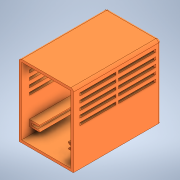
# Autodesk Inventor part: Back
Saved by Autodesk Inventor 2022 (Build 260153000, 153)
## iProperties
Created: 2022-01-12
Part Number: Back
Material: PLA Plastic
Document SubType Name: Modeling
Designer: chad
Density: 0.25 g/cm^3
Appearance: Generic(1)
Author: chad
Autodesk Inventor part; units mm, degrees
ref_plane "YZ Plane" through (0, 0, 0) normal (1, 0, 0) x (0, 1, 0)
ref_plane "XZ Plane" through (0, 0, 0) normal (0, 1, 0) x (-1, 0, 0)
ref_plane "XY Plane" through (0, 0, 0) normal (0, 0, 1) x (1, 0, 0)
sketch "Sketch1" plane through (0, 0, 0) normal (0, 0, 1) x (1, 0, 0)
  line L0 (0, 0) -> (42.2, 0)
  line L1 (42.2, 0) -> (42.2, 56.2)
  line L2 (42.2, 56.2) -> (0, 56.2)
  line L3 (0, 56.2) -> (0, 0)
  line L4 (17.1, 5) -> (25.1, 5) construction
  line L5 (17.1, 2.75) -> (25.1, 2.75)
  line L6 (25.1, 7.25) -> (17.1, 7.25)
  arc A0 (17.1, 7.25) -> (17.1, 2.75) centre (17.1, 5) ccw
  arc A1 (25.1, 2.75) -> (25.1, 7.25) centre (25.1, 5) ccw
  line L7 (21.1, 5) -> (29.1, 5) construction
  dimension "d0" = 42.2
  dimension "d1" = 56.2
  dimension "d2" = 4
  dimension "d3" = 0
  dimension "d4" = 4.5
  dimension "d91" = 21.1
  dimension "d92" = 5
  constraints: 18 end point, 4 point on circle, 4 tangent, 3 horizontal, 3 parallel, 2 centre point, 1 collinear, 1 midpoint, 1 perpendicular
  measures "d0" distance of L2.end L1.end
  measures "d1" distance of L1.end L0.end
  measures "d2" distance of L7.start L4.end
  measures "d3" distance between parallel lines of L4 L7
  measures "d4" diameter of A1
  measures "d91" distance from line of L7.start L3
  measures "d92" distance from line of L0 L7.start
extrude "Extrusion1" add sketch "Sketch1" along normal blind 68
shell "Shell1" thickness 2 removed faces 5 at (19.7667, 39.8833, 68) at (25.8125, 2.8658, 45.3333) at (16.3875, 7.1342, 45.3333) at (22.4333, 2.75, 22.6667) at (19.7667, 7.25, 22.6667)
sketch "Sketch3" plane through (42.2, 0, 0) normal (1, 0, 0) x (0, 0, -1)
  line L0 (-35, 49.2) -> (-62, 49.2)
  line L1 (-62, 49.2) -> (-62, 51.2)
  line L2 (-62, 51.2) -> (-35, 51.2)
  line L3 (-35, 51.2) -> (-35, 49.2)
  line L4 (-35, 44.2) -> (-62, 44.2)
  line L5 (-62, 44.2) -> (-62, 46.2)
  line L6 (-62, 46.2) -> (-35, 46.2)
  line L7 (-35, 46.2) -> (-35, 44.2)
  line L8 (-35, 39.2) -> (-62, 39.2)
  line L9 (-62, 39.2) -> (-62, 41.2)
  line L10 (-62, 41.2) -> (-35, 41.2)
  line L11 (-35, 41.2) -> (-35, 39.2)
  line L12 (-35, 34.2) -> (-62, 34.2)
  line L13 (-62, 34.2) -> (-62, 36.2)
  line L14 (-35, 36.2) -> (-35, 34.2)
  line L15 (-62, 36.2) -> (-35, 36.2)
  line L16 (0, 56.2) -> (-68, 56.2) projected
  line L17 (-35, 29.2) -> (-62, 29.2)
  line L18 (-62, 29.2) -> (-62, 31.2)
  line L19 (-35, 31.2) -> (-35, 29.2)
  line L20 (-62, 31.2) -> (-35, 31.2)
  line L21 (-68, 0) -> (-68, 56.2) projected
  line L22 (-5, 49.2) -> (-33, 49.2)
  line L23 (-33, 49.2) -> (-33, 51.2)
  line L24 (-33, 51.2) -> (-5, 51.2)
  line L25 (-5, 51.2) -> (-5, 49.2)
  line L26 (-5, 44) -> (-33, 44)
  line L27 (-33, 44) -> (-33, 46)
  line L28 (-33, 46) -> (-5, 46)
  line L29 (-5, 46) -> (-5, 44)
  line L30 (-5, 39) -> (-33, 39)
  line L31 (-33, 39) -> (-33, 41)
  line L32 (-33, 41) -> (-5, 41)
  line L33 (-5, 41) -> (-5, 39)
  line L34 (-5, 34) -> (-33, 34)
  line L35 (-33, 34) -> (-33, 36)
  line L36 (-33, 36) -> (-5, 36)
  line L37 (-5, 36) -> (-5, 34)
  line L38 (-5, 29) -> (-33, 29)
  line L39 (-33, 29) -> (-33, 31)
  line L40 (-33, 31) -> (-5, 31)
  line L41 (-5, 31) -> (-5, 29)
  point P0 (0, 0)
  dimension "d11" = 27
  dimension "d12" = 2
  dimension "d13" = 27
  dimension "d14" = 2
  dimension "d15" = 3
  dimension "d16" = 27
  dimension "d17" = 2
  dimension "d18" = 27
  dimension "d19" = 2
  dimension "d20" = 3
  dimension "d21" = 3
  dimension "d22" = 5
  dimension "d23" = 27
  dimension "d24" = 2
  dimension "d25" = 3
  dimension "d47" = 6
  dimension "d48" = 6
  dimension "d49" = 6
  dimension "d50" = 6
  dimension "d51" = 6
  dimension "d74" = 28
  dimension "d75" = 2
  dimension "d76" = 5
  dimension "d77" = 2
  dimension "d78" = 28
  dimension "d79" = 2
  dimension "d80" = 28
  dimension "d81" = 2
  dimension "d82" = 28
  dimension "d83" = 2
  dimension "d84" = 28
  dimension "d85" = 2
  dimension "d100" = 2
  dimension "d101" = 2
  constraints: 80 end point, 20 parallel, 10 horizontal, 10 perpendicular, 2 point on line
  measures "d11" distance of L1.end L2.end
  measures "d12" distance of L0.end L1.end
  measures "d13" distance of L5.end L7.start
  measures "d14" distance of L4.end L5.end
  measures "d15" distance between parallel lines of L6 L0
  measures "d16" distance of L9.end L10.end
  measures "d17" distance of L8.end L9.end
  measures "d18" distance of L13.end L14.start
  measures "d19" distance of L12.end L13.end
  measures "d20" distance between parallel lines of L15 L8
  measures "d21" distance between parallel lines of L10 L4
  measures "d22" distance between parallel lines of L2 L16
  measures "d23" distance of L20.start L19.start
  measures "d24" distance of L17.end L20.start
  measures "d25" distance between parallel lines of L20 L12
  measures "d47" distance between parallel lines of L18 L21
  measures "d48" distance between parallel lines of L13 L21
  measures "d49" distance between parallel lines of L9 L21
  measures "d50" distance between parallel lines of L5 L21
  measures "d51" distance between parallel lines of L1 L21
  measures "d74" distance of L23.end L24.end
  measures "d75" distance of L22.end L23.end
  measures "d76" distance between parallel lines of L24 L16
  measures "d77" distance from line of L22.end L3
  measures "d78" distance of L27.end L28.end
  measures "d79" distance of L26.end L27.end
  measures "d80" distance of L31.end L32.end
  measures "d81" distance of L30.end L31.end
  measures "d82" distance of L35.end L36.end
  measures "d83" distance of L34.end L35.end
  measures "d84" distance of L39.end L40.end
  measures "d85" distance of L38.end L39.end
  measures "d100" distance between parallel lines of L7 L27
  measures "d101" distance between parallel lines of L11 L31
sketch "Sketch8" plane through (0, 0, 0) normal (-1, 0, 0) x (0, 0, 1)
  line L0 (62, 49) -> (35, 49)
  line L1 (35, 49) -> (35, 51)
  line L2 (35, 51) -> (62, 51)
  line L3 (62, 51) -> (62, 49)
  line L4 (62, 44) -> (35, 44)
  line L5 (35, 44) -> (35, 46)
  line L6 (62, 46) -> (62, 44)
  line L7 (35, 46) -> (62, 46)
  line L8 (62, 39) -> (35, 39)
  line L9 (35, 39) -> (35, 41)
  line L10 (35, 41) -> (62, 41)
  line L11 (62, 41) -> (62, 39)
  line L12 (62, 34) -> (35, 34)
  line L13 (35, 34) -> (35, 36)
  line L14 (62, 36) -> (62, 34)
  line L15 (35, 36) -> (62, 36)
  line L16 (62, 31) -> (62, 29)
  line L17 (62, 29) -> (35, 29)
  line L18 (35, 31) -> (62, 31)
  line L19 (35, 29) -> (35, 31)
  line L20 (68, 56.2) -> (68, 0) projected
  line L21 (5, 49.2) -> (33, 49.2)
  line L22 (33, 49.2) -> (33, 51.2)
  line L23 (33, 51.2) -> (5, 51.2)
  line L24 (5, 51.2) -> (5, 49.2)
  line L25 (0, 56.2) -> (68, 56.2) projected
  line L26 (5, 44.2) -> (33, 44.2)
  line L27 (33, 44.2) -> (33, 46.2)
  line L28 (33, 46.2) -> (5, 46.2)
  line L29 (5, 46.2) -> (5, 44.2)
  line L30 (5, 39.2) -> (33, 39.2)
  line L31 (33, 39.2) -> (33, 41.2)
  line L32 (33, 41.2) -> (5, 41.2)
  line L33 (5, 41.2) -> (5, 39.2)
  line L34 (5, 34) -> (33, 34)
  line L35 (33, 34) -> (33, 36)
  line L36 (33, 36) -> (5, 36)
  line L37 (5, 36) -> (5, 34)
  line L38 (5, 29) -> (33, 29)
  line L39 (33, 29) -> (33, 31)
  line L40 (33, 31) -> (5, 31)
  line L41 (5, 31) -> (5, 29)
  point P0 (0, 0)
  point P1 (0, 0)
  dimension "d26" = 27
  dimension "d27" = 2
  dimension "d28" = 27
  dimension "d29" = 2
  dimension "d30" = 3
  dimension "d31" = 27
  dimension "d32" = 2
  dimension "d33" = 27
  dimension "d34" = 2
  dimension "d35" = 3
  dimension "d36" = 3
  dimension "d38" = 27
  dimension "d39" = 2
  dimension "d40" = 3
  dimension "d52" = 6
  dimension "d53" = 6
  dimension "d54" = 6
  dimension "d55" = 6
  dimension "d56" = 6
  dimension "d57" = 28
  dimension "d58" = 2
  dimension "d59" = 5
  dimension "d60" = 28
  dimension "d61" = 2
  dimension "d62" = 3
  dimension "d63" = 2
  dimension "d64" = 2
  dimension "d65" = 28
  dimension "d66" = 2
  dimension "d67" = 3
  dimension "d68" = 28
  dimension "d69" = 2
  dimension "d70" = 28
  dimension "d71" = 2
  constraints: 80 end point, 20 parallel, 10 horizontal, 10 perpendicular
  measures "d26" distance of L1.end L2.end
  measures "d27" distance of L0.end L1.end
  measures "d28" distance of L5.end L6.start
  measures "d29" distance of L4.end L5.end
  measures "d30" distance between parallel lines of L7 L0
  measures "d31" distance of L9.end L10.end
  measures "d32" distance of L8.end L9.end
  measures "d33" distance of L13.end L14.start
  measures "d34" distance of L12.end L13.end
  measures "d35" distance between parallel lines of L15 L8
  measures "d36" distance between parallel lines of L10 L4
  measures "d38" distance of L18.start L16.start
  measures "d39" distance of L17.end L18.start
  measures "d40" distance between parallel lines of L18 L12
  measures "d52" distance between parallel lines of L3 L20
  measures "d53" distance between parallel lines of L6 L20
  measures "d54" distance between parallel lines of L11 L20
  measures "d55" distance between parallel lines of L14 L20
  measures "d56" distance between parallel lines of L16 L20
  measures "d57" distance of L23.end L22.end
  measures "d58" distance of L22.end L21.end
  measures "d59" distance between parallel lines of L23 L25
  measures "d60" distance of L28.end L27.end
  measures "d61" distance of L27.end L26.end
  measures "d62" distance between parallel lines of L28 L21
  measures "d63" distance between parallel lines of L22 L1
  measures "d64" distance between parallel lines of L27 L5
  measures "d65" distance of L32.end L31.end
  measures "d66" distance of L31.end L30.end
  measures "d67" distance between parallel lines of L32 L26
  measures "d68" distance of L36.end L35.end
  measures "d69" distance of L35.end L34.end
  measures "d70" distance of L40.end L39.end
  measures "d71" distance of L39.end L38.end
sketch "Sketch9" plane through (0, 0, 0) normal (-1, 0, 0) x (0, 0, 1)
  point P0 (0, 0)
extrude "Extrusion4" cut sketch "Sketch8" against normal blind 2
extrude "Extrusion5" cut sketch "Sketch3" against normal blind 2
fillet "Fillet3" radius 1 10 edges at (42.2, 50.2, 62) (42.2, 45.2, 62) (42.2, 40.2, 62) (42.2, 35.2, 62) (42.2, 30.2, 62) (42.2, 50.2, 5) (42.2, 45, 5) (42.2, 40, 5) (42.2, 35, 5) (42.2, 30, 5)
fillet "Fillet4" radius 1 10 edges at (0, 50.2, 5) (0, 45.2, 5) (0, 40.2, 5) (0, 35, 5) (0, 30, 5) (0, 50, 62) (0, 45, 62) (0, 40, 62) (0, 35, 62) (0, 30, 62)
fillet "Fillet5" radius 2 5 edges at (42.2, 56.2, 34) (0, 56.2, 34) (21.1, 56.2, 0) (42.2, 28.1, 0) (0, 28.1, 0)
sketch "Sketch11" plane through (0, 0, 0) normal (0, 0, -1) x (-1, 0, 0)
  line L0 (-2, 54.2) -> (-2, 2) projected
  line L1 (-40.2, 2) -> (-40.2, 54.2) projected
  line L2 (-25.1, 5) -> (-17.1, 5) construction
  line L3 (-25.1, 2) -> (-17.1, 2)
  line L4 (-17.1, 8) -> (-25.1, 8)
  arc A0 (-25.1, 8) -> (-25.1, 2) centre (-25.1, 5) ccw
  arc A1 (-17.1, 2) -> (-17.1, 8) centre (-17.1, 5) ccw
  line L5 (0, 0) -> (-42.2, 0) projected
  point P0 (-21.1, 5)
  dimension "d93" = 38.2
  dimension "d94" = 4
  dimension "d95" = 6
  dimension "d96" = 19.1
  dimension "d118" = 5
  constraints: 8 end point, 4 point on circle, 4 tangent, 2 centre point, 1 horizontal, 1 midpoint, 1 parallel
  measures "d93" distance between parallel lines of L0 L1
  measures "d94" distance of point (-21.1, 5) L2.end
  measures "d95" diameter of A1
  measures "d96" distance from line of point (-21.1, 5) L1
  measures "d118" distance from line of L5 point (-21.1, 5)
extrude "Extrusion6" cut sketch "Sketch11" against normal blind 1
fillet "Fillet6" radius 1 4 edges at (14.1, 5, 0) (21.1, 2, 0) (28.1, 5, 0) (21.1, 8, 0) inverted yes
sketch "Sketch12" plane through (0, 0, 0) normal (-1, 0, 0) x (0, 0, 1)
  line L0 (2, 54.2) -> (2, 2) projected
  line L1 (68, 54.2) -> (68, 0) projected
  line L2 (2, 8) -> (62, 8)
  line L3 (62, 8) -> (62, 9.5)
  line L4 (62, 9.5) -> (2, 9.5)
  line L5 (2, 9.5) -> (2, 8)
  line L6 (2, 11.4) -> (62, 11.4)
  line L7 (62, 11.4) -> (62, 12.9)
  line L8 (62, 12.9) -> (2, 12.9)
  line L9 (2, 12.9) -> (2, 11.4)
  line L10 (2, 2) -> (68, 2) projected
  line L11 (62, 9.5) -> (2, 9.5)
  line L12 (2, 9.5) -> (2, 11.4)
  line L13 (2, 11.4) -> (62, 11.4)
  line L14 (62, 11.4) -> (62, 9.5)
  line L15 (2, 9.5) -> (62, 9.5)
  line L16 (62, 9.5) -> (62, 11.4)
  line L17 (62, 11.4) -> (2, 11.4)
  line L18 (2, 11.4) -> (2, 9.5)
  line L19 (2, 9.5) -> (62, 9.5)
  line L20 (62, 9.5) -> (62, 11.4)
  line L21 (62, 11.4) -> (2, 11.4)
  line L22 (2, 11.4) -> (2, 9.5)
  point P0 (0, 0)
  point P1 (2, 9.5)
  dimension "d102" = 66
  dimension "d103" = 60
  dimension "d104" = 1.5
  dimension "d105" = 1.5
  dimension "d106" = 1.9
  dimension "d107" = 6
  dimension "d121" = 60
  constraints: 40 end point, 10 parallel, 5 horizontal, 5 perpendicular, 2 point on line
  measures "d102" distance between parallel lines of L0 L1
  measures "d103" distance of L4.end L3.end
  measures "d104" distance of L3.end L2.end
  measures "d105" distance of L7.end L6.end
  measures "d106" distance between parallel lines of L4 L6
  measures "d107" distance between parallel lines of L10 L2
  measures "d121" distance between parallel lines of L0 L7
sketch "Sketch13" plane through (42.2, 0, 68) normal (1, 0, 0) x (0, 0, -1)
  line L0 (6, 54.2) -> (6, 2)
  line L1 (68, 54.2) -> (68, 0)
  line L2 (6, 8) -> (66, 8)
  line L3 (66, 8) -> (66, 9.5)
  line L4 (66, 9.5) -> (6, 9.5)
  line L5 (6, 9.5) -> (6, 8)
  line L6 (6, 11.4) -> (66, 11.4)
  line L7 (66, 11.4) -> (66, 12.9)
  line L8 (66, 12.9) -> (6, 12.9)
  line L9 (6, 12.9) -> (6, 11.4)
  line L10 (6, 2) -> (68, 2)
  line L11 (66, 9.2488) -> (6, 9.2488)
  line L12 (6, 9.2488) -> (6, 11.7488)
  line L13 (6, 11.7488) -> (66, 11.7488)
  line L14 (66, 11.7488) -> (66, 9.2488)
  point P0 (68, 0)
  point P1 (0, 0)
  point P2 (6, 9.5)
  point P3 (6, 12.9)
  point P4 (6, 11.7488)
  point P5 (6, 9.2488)
  dimension "d108" = 62
  dimension "d109" = 60
  dimension "d110" = 1.5
  dimension "d111" = 1.5
  dimension "d113" = 6
  dimension "d119" = 2
  dimension "d120" = 2
  dimension "d123" = 60
  dimension "d124" = 2
  dimension "d125" = 2.5
  constraints: 30 end point, 6 parallel, 3 horizontal, 3 perpendicular, 2 point on line
  measures "d108" distance between parallel lines of L0 L1
  measures "d109" distance of L4.end L3.end
  measures "d110" distance of L3.end L2.end
  measures "d111" distance of L7.end L6.end
  measures "d113" distance between parallel lines of L10 L2
  measures "d119" distance between parallel lines of L1 L7
  measures "d120" distance between parallel lines of L1 L3
  measures "d123" distance between parallel lines of L14 L12
  measures "d124" distance between parallel lines of L1 L14
  measures "d125" distance between parallel lines of L11 L13
extrude "Extrusion7" add sketch "Sketch13" against normal blind 10 contours L8 L7 L13 L0 | L13 L7 L6 L0 | L4 L3 L11 L0 | L11 L3 L2 L0
extrude "Extrusion8" add sketch "Sketch12" against normal blind 10 contours L8 L7 L6 L0 | L4 L3 L2 L0
fillet "Fillet7" radius 1.5 4 edges at (32.2, 11.4, 32) (32.2, 9.5, 32) (10, 11.4, 32) (10, 9.5, 32)
extrude "Extrusion9" add sketch "Sketch13" against normal blind 4 contours L13 L7 L6 L0 | L6 L14 L4 L0 | L4 L3 L11 L0
extrude "Extrusion10" add sketch "Sketch12" against normal blind 4 contours L6 L14 L4 L0
equation "\"d91\" = 0.5 * d0"
equation "\"d13\" = d11"
equation "\"d16\" = d11"
equation "\"d18\" = d11"
equation "\"d23\" = d11"
equation "\"d100\" = d77"
equation "\"d101\" = d77"
equation "\"d96\" = 0.5 * d93"
body "Solid1"
